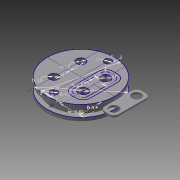
# Autodesk Inventor part: Winch
Saved by Autodesk Inventor 2014 SP1 (Build 180222100, 222)
## iProperties
Created: 2014-12-23
Part Number: Winch
Material: Generic
Document SubType Name: Modeling
Designer: Erin
Density: 1 g/cm^3
Appearance: Default
Author: Erin
Autodesk Inventor part; units mm, degrees
ref_plane "YZ Plane" through (0, 0, 0) normal (1, 0, 0) x (0, 1, 0)
ref_plane "XZ Plane" through (0, 0, 0) normal (0, 1, 0) x (-1, 0, 0)
sketch "Sketch1" plane through (0, 0, 0) normal (0, 0, 1) x (1, 0, 0)
  circle A0 centre (0, 0) radius 15
  circle A1 centre (-6, 6) radius 1.9
  circle A2 centre (6, 6) radius 1.9
  line L0 (-18.6167, 6) -> (18.2218, 6) construction
  line L1 (-15, 0) -> (15, 0) construction
  circle A3 centre (-5, -6) radius 2.05
  circle A4 centre (5, -6) radius 2.05
  line L2 (-13.6961, -6) -> (14.631, -6) construction
  line L3 (0, 15) -> (0, -15) construction
  line L4 (-6.05, -2.95) -> (6.05, -2.95)
  line L5 (8.05, -4.95) -> (8.05, -7.05)
  line L6 (6.05, -9.05) -> (-6.05, -9.05)
  line L7 (-8.05, -7.05) -> (-8.05, -4.95)
  arc A5 (-6.05, -2.95) -> (-8.05, -4.95) centre (-6.05, -4.95) ccw
  arc A6 (8.05, -4.95) -> (6.05, -2.95) centre (6.05, -4.95) ccw
  arc A7 (6.05, -9.05) -> (8.05, -7.05) centre (6.05, -7.05) ccw
  arc A8 (-8.05, -7.05) -> (-6.05, -9.05) centre (-6.05, -7.05) ccw
  line L8 (6.05, -1.75) -> (-6.05, -1.75)
  arc A9 (-6.05, -1.75) -> (-9.25, -4.95) centre (-6.05, -4.95) ccw
  line L9 (-9.25, -4.95) -> (-9.25, -7.05)
  arc A10 (-9.25, -7.05) -> (-6.05, -10.25) centre (-6.05, -7.05) ccw
  line L10 (-6.05, -10.25) -> (6.05, -10.25)
  arc A11 (6.05, -10.25) -> (9.25, -7.05) centre (6.05, -7.05) ccw
  line L11 (9.25, -7.05) -> (9.25, -4.95)
  arc A12 (9.25, -4.95) -> (6.05, -1.75) centre (6.05, -4.95) ccw
  circle A13 centre (-12, 0) radius 1.5
  circle A14 centre (12, 0) radius 1.5
  dimension "d0" = 3.8
  dimension "d1" = 3.8
  dimension "d2" = 30
  dimension "d3" = 4.1
  dimension "d4" = 4.1
  dimension "d5" = 6
  dimension "d6" = 6
  dimension "d7" = 6
  dimension "d8" = 6
  dimension "d9" = 5
  dimension "d10" = 5
  dimension "d11" = 1
  dimension "d12" = 1
  dimension "d13" = 1
  dimension "d14" = 1
  dimension "d15" = 2
  dimension "d16" = 1.2
  dimension "d61" = 3
  dimension "d62" = 1.5
  dimension "d63" = 3
  dimension "d64" = 1.5
  constraints: 24 end point, 20 point on circle, 15 centre point, 8 tangent, 6 parallel, 6 point on line, 3 equal radius, 3 horizontal, 3 perpendicular, 1 coincident, 1 vertical, 7 other
  measures "d0" diameter of A1
  measures "d1" diameter of A2
  measures "d2" diameter of A0
  measures "d3" diameter of A3
  measures "d4" diameter of A4
  measures "d5" distance between parallel lines of L2 L1
  measures "d6" distance between parallel lines of L0 L1
  measures "d7" distance from line of L3 A1.centre
  measures "d8" distance from line of A2.centre L3
  measures "d9" distance from line of A3.centre L3
  measures "d10" distance from line of A4.centre L3
  measures "d11" distance edge to line of A3 L6
  measures "d12" distance edge to line of A3 L7
  measures "d13" distance edge to line of A4 L5
  measures "d14" distance edge to line of A3 L4
  measures "d15" radius of A5
  measures "d16" distance between parallel lines of L4 L8
  measures "d61" diameter of A13
  measures "d63" diameter of A14
extrude "Extrusion1" add sketch "Sketch1" along normal blind 2 contours A0 | A1 | A2 | A3 | A4 | L4 A6 L5 A7 L6 A8 L7 A5 | A12 L11 A11 L10 A10 L9 A9 L8 | A13 | A14
ref_plane "Work Plane1" through (0, 0, 2) normal (0, 0, 1) x (1, 0, 0)
sketch "Sketch2" plane through (0, 0, 2) normal (0, 0, 1) x (1, 0, 0)
  circle A0 centre (0, 0) radius 13
  dimension "d20" = 26
  constraints: 1 centre point, 1 coincident
  measures "d20" diameter of A0
extrude "Extrusion2" add sketch "Sketch2" along normal blind 3
ref_plane "Work Plane2" through (0, 0, 5) normal (0, 0, 1) x (1, 0, 0)
sketch "Sketch3" plane through (0, 0, 5) normal (0, 0, 1) x (1, 0, 0)
  circle A0 centre (0, 0) radius 15
  circle A1 centre (-5, -6) radius 2.05 projected
  circle A2 centre (5, -6) radius 2.05 projected
  line L0 (0.3008, -8.6363) -> (0.2992, -3.372)
  line L1 (9.6992, -3.3637) -> (9.7008, -8.628)
  line L2 (9.7, -5.9959) -> (0.3, -6.0041) construction
  line L3 (9.7008, -8.628) -> (5.0046, -11.2)
  line L4 (5.0046, -11.2) -> (0.3008, -8.6363)
  line L5 (9.6992, -3.3637) -> (4.9954, -0.8)
  line L6 (4.9954, -0.8) -> (0.2992, -3.372)
  line L7 (9.7008, -8.628) -> (0.3008, -8.6363) construction
  line L8 (5.0046, -11.2) -> (4.9954, -0.8) construction
  dimension "d24" = 30
  dimension "d35" = 9.4
  dimension "d36" = 10.4
  constraints: 18 end point, 4 parallel, 3 midpoint, 2 coincident, 1 centre point, 1 perpendicular
  measures "d24" diameter of A0
  measures "d35" distance between parallel lines of L0 L1
  measures "d36" distance of L5.end L3.end
extrude "Extrusion3" add sketch "Sketch3" along normal blind 1.5 contours A0 | A1 | A2 | L0 L6 L5 L1 L3 L4
extrude "Extrusion5" cut sketch "Sketch1" along normal blind 6 contours A1 | A2
extrude "Extrusion6" [suppressed]
extrude "Extrusion7" cut sketch "Sketch1" along normal blind 7 contours A3 | A4
sketch "Sketch4" plane through (0, 0, 6.5) normal (0, 0, 1) x (1, 0, 0)
  circle A0 centre (0, 0) radius 12.5
  line L0 (9.2, -5.9963) -> (0.8, -6.0037) construction
  line L1 (9.2, -8.792) -> (0.8, -8.7993) construction
  line L2 (5.0041, -10.7) -> (4.9959, -1.3) construction
  circle A1 centre (5, -6) radius 2
  line L3 (5, 10) -> (5, 0) construction
  line L4 (4.7529, -0.9787) -> (8.9779, -3.418)
  line L5 (8.9779, -3.418) -> (8.9779, -8.8672)
  line L6 (8.9779, -8.8672) -> (5, -11.1639)
  line L7 (5, -11.1639) -> (0.5279, -8.582)
  line L8 (0.5279, -8.582) -> (0.5279, -3.418)
  line L9 (0.5279, -3.418) -> (4.7529, -0.9787)
  line L10 (9.5779, -3.0716) -> (4.7529, -0.2859)
  line L11 (4.7529, -0.2859) -> (-0.0721, -3.0716)
  line L12 (-0.0721, -3.0716) -> (-0.0721, -8.9284)
  line L13 (-0.0721, -8.9284) -> (5, -11.8567)
  line L14 (5, -11.8567) -> (9.5779, -9.2137)
  line L15 (9.5779, -9.2137) -> (9.5779, -3.0716)
  point P0 (5, -6)
  point P1 (5, 5)
  dimension "d37" = 25
  dimension "d39" = 9.4
  dimension "d65" = 8.45
  dimension "d66" = 0.6
  constraints: 32 end point, 2 centre point, 1 midpoint, 1 parallel, 1 perpendicular, 6 other
  measures "d37" diameter of A0
  measures "d39" distance of L2.end L2.start
  measures "d65" distance between parallel lines of L5 L8
  measures "d66" distance between parallel lines of L10 L4
extrude "Extrusion8" cut sketch "Sketch4" against normal blind 3 contours L13 L12 L11 L10 L15 A0 L5 L4 L9 L8 L7 L6 | A0 L6 L5 L15 L14 L13 | L6 L7 L8 L9 L4 L5 A0 | A0 L5 L6
mirror "Mirror1" about plane through (0, 0, 0) normal (1, 0, 0) of "Extrusion8"
fillet "Fillet1" radius 1.5 1 edges at (-13, 0, 2)
sketch "Sketch5" plane through (0, 0, 0) normal (0, 0, 1) x (1, 0, 0)
  circle A0 centre (-5.0256, -19.7665) radius 2.05
  circle A1 centre (4.9744, -19.7665) radius 2.05
  line L0 (-6.0756, -16.7165) -> (6.0244, -16.7165)
  line L1 (8.0244, -18.7165) -> (8.0244, -20.8165)
  line L2 (6.0244, -22.8165) -> (-6.0756, -22.8165)
  line L3 (-8.0756, -20.8165) -> (-8.0756, -18.7165)
  arc A2 (-6.0756, -16.7165) -> (-8.0756, -18.7165) centre (-6.0756, -18.7165) ccw
  arc A3 (8.0244, -18.7165) -> (6.0244, -16.7165) centre (6.0244, -18.7165) ccw
  arc A4 (6.0244, -22.8165) -> (8.0244, -20.8165) centre (6.0244, -20.8165) ccw
  arc A5 (-8.0756, -20.8165) -> (-6.0756, -22.8165) centre (-6.0756, -20.8165) ccw
  line L4 (6.0244, -16.1165) -> (-6.0756, -16.1165)
  arc A6 (-6.0756, -16.1165) -> (-8.6756, -18.7165) centre (-6.0756, -18.7165) ccw
  line L5 (-8.6756, -18.7165) -> (-8.6756, -20.8165)
  arc A7 (-8.6756, -20.8165) -> (-6.0756, -23.4165) centre (-6.0756, -20.8165) ccw
  line L6 (-6.0756, -23.4165) -> (6.0244, -23.4165)
  arc A8 (6.0244, -23.4165) -> (8.6244, -20.8165) centre (6.0244, -20.8165) ccw
  line L7 (8.6244, -20.8165) -> (8.6244, -18.7165)
  arc A9 (8.6244, -18.7165) -> (6.0244, -16.1165) centre (6.0244, -18.7165) ccw
  dimension "d44" = 4.1
  dimension "d45" = 4.1
  dimension "d46" = 1
  dimension "d47" = 1
  dimension "d48" = 1
  dimension "d49" = 1
  dimension "d50" = 2
  dimension "d51" = 0.6
  constraints: 16 end point, 16 point on circle, 10 centre point, 8 tangent, 4 parallel, 3 equal radius, 2 perpendicular, 1 horizontal, 7 other
  measures "d44" diameter of A0
  measures "d45" diameter of A1
  measures "d46" distance edge to line of A0 L2
  measures "d47" distance edge to line of A0 L3
  measures "d48" distance edge to line of A1 L1
  measures "d49" distance edge to line of A0 L0
  measures "d50" radius of A2
  measures "d51" distance between parallel lines of L0 L4
extrude "Extrusion9" add sketch "Sketch5" along normal blind 0.8 contours L0 A3 L1 A4 L2 A5 L3 A2
extrude "Extrusion10" cut sketch "Sketch1" along normal through all contours A13 | A14
sketch "Sketch6" plane through (0, 0, 6.5) normal (0, 0, 1) x (1, 0, 0)
  circle A0 centre (0, 0) radius 15 projected
  circle A1 centre (0, 0) radius 1.825
  dimension "d67" = 3.65
  constraints: 1 centre point, 1 coincident
  measures "d67" diameter of A1
extrude "Extrusion11" cut sketch "Sketch6" against normal blind 1 contours A1
equation "\"d0\" = rivet + sp"
equation "\"d1\" = rivet + sp"
equation "\"d3\" = screw + sp"
equation "\"d4\" = screw + sp"
equation "\"d16\" = 2 * sp"
equation "\"d66\" = sp"
equation "\"d44\" = d53 + d52"
equation "\"d45\" = d53 + d52"
equation "\"d51\" = d52"
equation "\"rivet\" = 3.2"
equation "\"sp\" = 0.6"
equation "\"screw\" = 3.5"
equation "\"d40\" = 0.6"
equation "\"d52\" = 0.6"
equation "\"d53\" = 3.5"
body "Solid1"
